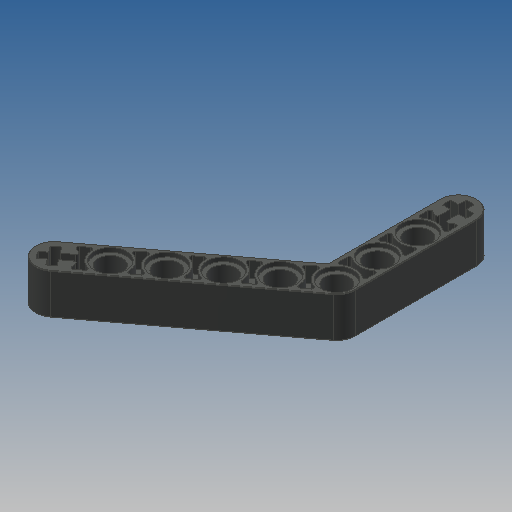
# Autodesk Inventor part: 6629-DkBluishGray
Saved by Autodesk Inventor 2022.2 (Build 262287010, 287A)
## iProperties
Created: 2012-03-21
Part Number: 6629-DkBluishGray
Document SubType Name: Modeling
Designer: D. Kohfeld
Density: 1.06 g/cm^3
Material: ABS Plastic
Appearance: DkBluishGray
Mass: 2.31201 g
Surface Area: 38.6111 cm^2
Volume: 2.18114 cm^3
Author: D. Kohfeld
Autodesk Inventor part; units mm, degrees
ref_plane "YZ Plane" through (0, 0, 0) normal (1, 0, 0) x (0, 1, 0)
ref_plane "XZ Plane" through (0, 0, 0) normal (0, 1, 0) x (-1, 0, 0)
ref_plane "XY Plane" through (0, 0, 0) normal (0, 0, 1) x (1, 0, 0)
sketch "Sketch1" plane through (0, 0, 0) normal (0, 0, 1) x (1, 0, 0)
  line L0 (-3.6, 24) -> (-3.6, 0)
  arc A0 (3.6, 24) -> (-3.6, 24) centre (0, 24) ccw
  circle A1 centre (0, 24) radius 3.2 construction
  circle A2 centre (0, 24) radius 2.4 construction
  line L1 (2.8, 21.7373) -> (2.8, 18.2627)
  line L2 (-2.8, 21.7373) -> (-2.8, 18.2627)
  arc A3 (-2.8, 21.7373) -> (2.8, 21.7373) centre (0, 24) ccw
  arc A4 (2.8, 18.2627) -> (-2.8, 18.2627) centre (0, 16) ccw
  circle A5 centre (0, 16) radius 3.2
  circle A6 centre (0, 16) radius 2.4
  line L3 (-0.8, 20.49) -> (-0.8, 23.2)
  line L4 (-0.8, 23.2) -> (-2.2627, 23.2)
  line L5 (-2.2627, 24.8) -> (-0.8, 24.8)
  line L6 (-0.8, 24.8) -> (-0.8, 26.2627)
  line L7 (0.8, 26.2627) -> (0.8, 24.8)
  line L8 (0.8, 24.8) -> (2.2627, 24.8)
  line L9 (2.2627, 23.2) -> (0.8, 23.2)
  line L10 (0.8, 23.2) -> (0.8, 20.49)
  arc A7 (-2.2627, 24.8) -> (-2.2627, 23.2) centre (0, 24) ccw
  arc A8 (0.8, 26.2627) -> (-0.8, 26.2627) centre (0, 24) ccw
  arc A9 (2.2627, 23.2) -> (2.2627, 24.8) centre (0, 24) ccw
  line L11 (3.6, 0) -> (3.6, 24)
  arc A10 (-3.6, 0) -> (3.6, 0) centre (0, 0) ccw
  line L12 (2.16, -2.88) -> (-29.84, -26.8801)
  arc A11 (-34.16, -21.1201) -> (-29.84, -26.8801) centre (-32, -24.0001) ccw
  line L13 (-34.16, -21.1201) -> (-3.6, 1.8)
  circle A12 centre (-6.4, -4.8) radius 3.2
  circle A13 centre (-12.8, -9.6) radius 3.2
  circle A14 centre (-19.2, -14.4) radius 3.2
  circle A15 centre (-25.6, -19.2) radius 3.2
  line L14 (-32, -24.0001) -> (-25.6, -19.2) construction
  line L15 (-25.6, -19.2) -> (-19.2, -14.4) construction
  line L16 (-19.2, -14.4) -> (-12.8, -9.6) construction
  line L17 (-12.8, -9.6) -> (-6.4, -4.8) construction
  line L18 (-6.4, -4.8) -> (0, 0) construction
  line L19 (0, 24) -> (0, 16) construction
  line L20 (0, 16) -> (0, 8) construction
  line L21 (0, 8) -> (0, 0) construction
  circle A16 centre (0, 8) radius 3.2
  circle A17 centre (0, 8) radius 2.4
  circle A18 centre (0, 0) radius 3.2
  circle A19 centre (0, 0) radius 2.4
  circle A20 centre (-6.4, -4.8) radius 2.4
  circle A21 centre (-12.8, -9.6) radius 2.4
  circle A22 centre (-19.2, -14.4) radius 2.4
  circle A23 centre (-25.6, -19.2) radius 2.4
  circle A24 centre (-32, -24.0001) radius 2.4 construction
  circle A25 centre (-32, -24.0001) radius 3.2 construction
  line L22 (2.8, 13.7373) -> (2.8, 10.2627)
  line L23 (-2.8, 13.7373) -> (-2.8, 10.2627)
  arc A26 (-2.8, 13.7373) -> (2.8, 13.7373) centre (0, 16) ccw
  arc A27 (2.8, 10.2627) -> (-2.8, 10.2627) centre (0, 8) ccw
  line L24 (2.8, 5.7373) -> (2.8, 2.2627)
  line L25 (-2.8, 5.7373) -> (-2.8, 2.2627)
  arc A28 (-2.8, 5.7373) -> (2.8, 5.7373) centre (0, 8) ccw
  arc A29 (2.8, 2.2627) -> (-2.8, 2.2627) centre (0, 0) ccw
  line L26 (-3.4902, 0.8823) -> (-6.2698, -1.2024)
  line L27 (-2.9098, -5.6824) -> (-0.1302, -3.5976)
  arc A30 (-2.9098, -5.6824) -> (-6.2698, -1.2024) centre (-6.4, -4.8) ccw
  arc A31 (-3.4902, 0.8823) -> (-0.1302, -3.5976) centre (0, 0) ccw
  line L28 (-9.8902, -3.9177) -> (-12.6698, -6.0024)
  line L29 (-9.3098, -10.4824) -> (-6.5302, -8.3977)
  arc A32 (-9.3098, -10.4824) -> (-12.6698, -6.0024) centre (-12.8, -9.6) ccw
  arc A33 (-9.8902, -3.9177) -> (-6.5302, -8.3977) centre (-6.4, -4.8) ccw
  line L30 (-16.2902, -8.7177) -> (-19.0698, -10.8024)
  line L31 (-15.7098, -15.2824) -> (-12.9302, -13.1977)
  arc A34 (-15.7098, -15.2824) -> (-19.0698, -10.8024) centre (-19.2, -14.4) ccw
  arc A35 (-16.2902, -8.7177) -> (-12.9302, -13.1977) centre (-12.8, -9.6) ccw
  line L32 (-22.6902, -13.5177) -> (-25.4698, -15.6024)
  line L33 (-22.1098, -20.0824) -> (-19.3302, -17.9977)
  arc A36 (-22.1098, -20.0824) -> (-25.4698, -15.6024) centre (-25.6, -19.2) ccw
  arc A37 (-22.6902, -13.5177) -> (-19.3302, -17.9977) centre (-19.2, -14.4) ccw
  line L34 (-29.0902, -18.3177) -> (-31.8698, -20.4024)
  line L35 (-28.5098, -24.8824) -> (-25.7302, -22.7977)
  arc A38 (-28.5098, -24.8824) -> (-31.8698, -20.4024) centre (-32, -24.0001) ccw
  arc A39 (-29.0902, -18.3177) -> (-25.7302, -22.7977) centre (-25.6, -19.2) ccw
  line L36 (-34.2901, -24.7177) -> (-33.12, -23.8401)
  line L37 (-33.12, -23.8401) -> (-33.9976, -22.6699)
  line L38 (-32.7176, -21.7099) -> (-31.84, -22.8801)
  line L39 (-31.84, -22.8801) -> (-29.672, -21.2541)
  line L40 (-33.3301, -25.9977) -> (-32.16, -25.1201)
  line L41 (-32.16, -25.1201) -> (-31.2823, -26.2902)
  line L42 (-30.0023, -25.3302) -> (-30.88, -24.1601)
  line L43 (-30.88, -24.1601) -> (-28.712, -22.5341)
  arc A40 (-32.7176, -21.7099) -> (-33.9976, -22.6699) centre (-32, -24.0001) ccw
  arc A41 (-34.2901, -24.7177) -> (-33.3301, -25.9977) centre (-32, -24.0001) ccw
  arc A42 (-31.2823, -26.2902) -> (-30.0023, -25.3302) centre (-32, -24.0001) ccw
  point P0 (-0.8, 12.49)
  point P1 (0.8, 12.49)
  point P2 (-0.8, 4.49)
  point P3 (0.8, 4.49)
  dimension "d32" = 7.2
  dimension "d49" = 6.4
  dimension "d50" = 4.8
  dimension "d52" = 0.8
  dimension "d62" = 1.6
  dimension "d76" = 8
  dimension "d77" = 8
  dimension "d78" = 4.8
  dimension "d81" = 8
  dimension "d86" = 0.8
  dimension "d89" = 8
  dimension "d94" = 1.6
  dimension "d95" = 1.6
  dimension "d96" = 1.6
  dimension "d97" = 53.13
  constraints: 88 end point, 71 point on circle, 43 centre point, 23 equal radius, 19 equal length, 16 coincident, 13 parallel, 8 perpendicular, 6 tangent, 5 collinear, 4 concentric, 4 vertical, 3 vertical alignment, 2 horizontal alignment, 2 point on line, 65 other
  measures "d32" diameter of A0
  measures "d49" diameter of A1
  measures "d50" diameter of A2
  measures "d52" distance between parallel lines of L0 L2
  measures "d62" distance between parallel lines of L10 L3
  measures "d76" distance of L17.end L18.end
  measures "d77" distance of L19.start L19.end
  measures "d78" diameter of A24
  measures "d81" distance of L2.start L23.start
  measures "d86" distance between parallel lines of L13 L26
  measures "d89" distance of L26.start L28.start
  measures "d94" distance between parallel lines of L36 L40
  measures "d95" distance between parallel lines of L43 L39
  measures "d96" distance between parallel lines of L38 L37
  measures "d97" angle of L11 L12
extrude "Extrusion1" add sketch "Sketch1" along normal mid plane 8 contours A0 L11 A10 A31 L26 L0 | L0 L26 A30 L27 A10 L12 A11 L13 | L26 A31 L0 | L0 A10 L27 A30 L26 | A5 | A12 | A13 | A14 | A15 | A16 | A18 | L22 A27 L23 A26 | L24 A29 L25 A28 | A33 L29 A32 L28 | A35 L31 A34 L30 | A37 L33 A36 L32
sketch "Sketch6" plane through (0, 0, 4) normal (0, 0, 1) x (1, 0, 0)
  circle A0 centre (0, 24) radius 3.2 projected
  line L0 (2.8, 21.7373) -> (2.8, 18.2627) projected
  arc A1 (-2.8, 21.7373) -> (2.8, 21.7373) centre (0, 24) ccw projected
  arc A2 (2.8, 18.2627) -> (-2.8, 18.2627) centre (0, 16) ccw projected
  line L1 (-2.8, 21.7373) -> (-2.8, 18.2627) projected
  circle A3 centre (0, 16) radius 3.2 projected
  circle A4 centre (0, 16) radius 3.1 projected
  line L2 (3.6, 24) -> (3.6, 0) projected
  line L3 (3.6, 0) -> (3.6, 24) projected
  line L4 (2.8, 13.7373) -> (2.8, 10.2627) projected
  arc A5 (2.8, 10.2627) -> (-2.8, 10.2627) centre (0, 8) ccw projected
  arc A6 (-2.8, 13.7373) -> (2.8, 13.7373) centre (0, 16) ccw projected
  line L5 (-2.8, 13.7373) -> (-2.8, 10.2627) projected
  circle A7 centre (0, 8) radius 3.2 projected
  arc A8 (-2.8, 5.7373) -> (2.8, 5.7373) centre (0, 8) ccw projected
  arc A9 (2.8, 2.2627) -> (-2.8, 2.2627) centre (0, 0) ccw projected
  line L6 (2.8, 5.7373) -> (2.8, 2.2627) projected
  line L7 (-2.8, 5.7373) -> (-2.8, 2.2627) projected
  circle A10 centre (0, 0) radius 3.2 projected
  arc A11 (-2.9098, -5.6824) -> (-6.2698, -1.2024) centre (-6.4, -4.8) ccw projected
  line L8 (-2.9098, -5.6824) -> (-0.1302, -3.5976) projected
  arc A12 (-3.4902, 0.8823) -> (-0.1302, -3.5976) centre (0, 0) ccw projected
  line L9 (-3.4902, 0.8823) -> (-6.2698, -1.2024) projected
  circle A13 centre (-6.4, -4.8) radius 3.2 projected
  arc A14 (-9.8902, -3.9177) -> (-6.5302, -8.3977) centre (-6.4, -4.8) ccw projected
  arc A15 (-9.3098, -10.4824) -> (-12.6698, -6.0024) centre (-12.8, -9.6) ccw projected
  line L10 (-9.3098, -10.4824) -> (-6.5302, -8.3977) projected
  line L11 (-9.8902, -3.9177) -> (-12.6698, -6.0024) projected
  circle A16 centre (-12.8, -9.6) radius 3.2 projected
  circle A17 centre (-19.2, -14.4) radius 3.2 projected
  circle A18 centre (-25.6, -19.2) radius 3.2 projected
  arc A19 (-22.1098, -20.0824) -> (-25.4698, -15.6024) centre (-25.6, -19.2) ccw projected
  arc A20 (-22.6902, -13.5177) -> (-19.3302, -17.9977) centre (-19.2, -14.4) ccw projected
  arc A21 (-15.7098, -15.2824) -> (-19.0698, -10.8024) centre (-19.2, -14.4) ccw projected
  arc A22 (-16.2902, -8.7177) -> (-12.9302, -13.1977) centre (-12.8, -9.6) ccw projected
  line L12 (-15.7098, -15.2824) -> (-12.9302, -13.1977) projected
  line L13 (-16.2902, -8.7177) -> (-19.0698, -10.8024) projected
  line L14 (-22.1098, -20.0824) -> (-19.3302, -17.9977) projected
  line L15 (-22.6902, -13.5177) -> (-25.4698, -15.6024) projected
extrude "Extrusion7" cut sketch "Sketch6" against normal blind 0.8 contours A3 | A4 | A7 | A10 | A13 | A16 | A17 | A18
extrude "Extrusion8" cut sketch "Sketch6" against normal blind 3.1 contours L4 A5 L5 A6 | A8 L6 A9 L7 | A11 L9 A12 L8 | A14 L10 A15 L11 | A19 L15 A20 L14 | A21 L13 A22 L12
mirror "Mirror1" about plane through (0, 0, 0) normal (0, 0, 1) of "Extrusion7", "Extrusion8"
fillet "Fillet2" radius 0.4 60 edges at (-2.8, 18.2627, 0) (-2.8, 21.7373, 0) (2.8, 18.2627, 0) (2.8, 21.7373, 0) (0.8, 20.49, 0) (-0.8, 20.49, 0) (-2.8, 13.7373, 2.45) (-2.8, 10.2627, 2.45) (2.8, 10.2627, 2.45) (2.8, 13.7373, 2.45) (-2.8, 5.7373, 2.45) (-2.8, 2.2627, 2.45) (2.8, 2.2627, 2.45) (2.8, 5.7373, 2.45) (-0.1302, -3.5976, 2.45) (-2.9098, -5.6824, 2.45) (-6.2698, -1.2024, 2.45) (-3.4902, 0.8823, 2.45) (-6.5302, -8.3977, 2.45) (-9.3098, -10.4824, 2.45) (-12.6698, -6.0024, 2.45) (-9.8902, -3.9177, 2.45) (-15.7098, -15.2824, 2.45) (-12.9302, -13.1977, 2.45) (-19.0698, -10.8024, 2.45) (-16.2902, -8.7177, 2.45) (-22.1098, -20.0824, 2.45) (-19.3302, -17.9977, 2.45) (-25.4698, -15.6024, 2.45) (-22.6902, -13.5177, 2.45) (-25.7302, -22.7977, 0) (-28.5098, -24.8824, 0) (-31.8698, -20.4024, 0) (-29.0902, -18.3177, 0) (2.8, 13.7373, -2.45) (2.8, 10.2627, -2.45) (-2.8, 10.2627, -2.45) (-2.8, 13.7373, -2.45) (-2.8, 5.7373, -2.45) (-2.8, 2.2627, -2.45) (2.8, 2.2627, -2.45) (2.8, 5.7373, -2.45) (-3.4902, 0.8823, -2.45) (-6.2698, -1.2024, -2.45) (-2.9098, -5.6824, -2.45) (-0.1302, -3.5976, -2.45) (-9.8902, -3.9177, -2.45) (-12.6698, -6.0024, -2.45) (-9.3098, -10.4824, -2.45) (-6.5302, -8.3977, -2.45) (-16.2902, -8.7177, -2.45) (-19.0698, -10.8024, -2.45) (-15.7098, -15.2824, -2.45) (-12.9302, -13.1977, -2.45) (-19.3302, -17.9977, -2.45) (-22.1098, -20.0824, -2.45) (-25.4698, -15.6024, -2.45) (-22.6902, -13.5177, -2.45) (-28.712, -22.5341, 0) (-29.672, -21.2541, 0)
fillet "Fillet2" radius 0.1 14 edges at (-3.6, 12.9, 4) (0, 27.6, 4) (3.6, 12, 4) (3.2199, -1.61, 4) (0, 27.6, -4) (-3.6, 12.9, -4) (3.2199, -1.61, -4) (3.6, 12, -4) (-34.88, -26.1601, 4) (-13.84, -14.88, 4) (-18.88, -9.66, 4) (-34.88, -26.1601, -4) (-18.88, -9.66, -4) (-13.84, -14.88, -4)
equation "\"lf\" = 0.1"
equation "\"tf\" = 0.4"
body "Solid1"
